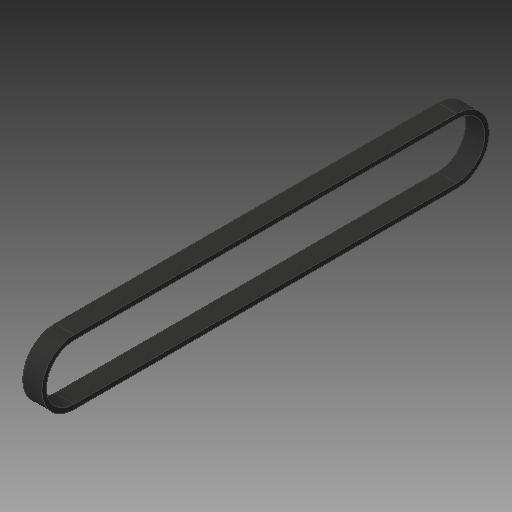
# Autodesk Inventor part: Belt 750
Saved by Autodesk Inventor 2019.4 (Build 234330000, 330)
## iProperties
Created: 2019-12-06
Part Number: Belt 750
Material: Rubber
Document SubType Name: Modeling
Designer: Mark
Density: 0.93 g/cm^3
Appearance: Rubber - Black
Mass: 37.5709 g
Surface Area: 278.303 cm^2
Volume: 40.3988 cm^3
Author: Mark
Autodesk Inventor part; units mm, degrees
ref_plane "YZ Plane" through (0, 0, 0) normal (1, 0, 0) x (0, 1, 0)
ref_plane "XZ Plane" through (0, 0, 0) normal (0, 1, 0) x (-1, 0, 0)
ref_plane "XY Plane" through (0, 0, 0) normal (0, 0, 1) x (1, 0, 0)
sketch "Sketch1" plane through (0, 0, 0) normal (1, 0, 0) x (0, 1, 0)
  line L0 (0, 150) -> (0, -150) construction
  line L1 (-23.875, 150) -> (-23.875, -150)
  line L2 (23.875, -150) -> (23.875, 150)
  arc A0 (23.875, 150) -> (-23.875, 150) centre (0, 150) ccw
  arc A1 (-23.875, -150) -> (23.875, -150) centre (0, -150) ccw
  line L3 (0, 0) -> (300, 0) construction
  line L4 (25.375, 150) -> (25.375, -150)
  arc A2 (-25.375, -150) -> (25.375, -150) centre (0, -150) ccw
  line L5 (-25.375, -150) -> (-25.375, 150)
  arc A3 (25.375, 150) -> (-25.375, 150) centre (0, 150) ccw
  line L6 (21.775, 150) -> (21.775, -150)
  arc A4 (-21.775, -150) -> (21.775, -150) centre (0, -150) ccw
  line L7 (-21.775, -150) -> (-21.775, 150)
  arc A5 (21.775, 150) -> (-21.775, 150) centre (0, 150) ccw
  dimension "d0" = 150
  dimension "d1" = 90
  dimension "d2" = 47.75
  dimension "d3" = 1.5
  dimension "d4" = 2.1
  constraints: 18 end point, 12 point on circle, 6 centre point, 4 tangent, 3 parallel, 1 horizontal, 1 midpoint, 1 perpendicular, 1 vertical, 6 other
  measures "d0" distance of L3.start L0.end
  measures "d1" angle of L0 L3
  measures "d2" diameter of A1
  measures "d3" distance between parallel lines of L2 L4
  measures "d4" distance between parallel lines of L2 L6
extrude "Extrusion1" add sketch "Sketch1" along normal blind 15 contours A0 L2 A1 L1 | L4 A2 L5 A3
body "Solid1"
